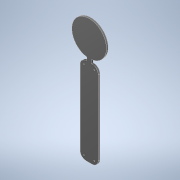
# Autodesk Inventor part: Body1
Saved by Autodesk Inventor 2022 (Build 260153000, 153)
## iProperties
Created: 2022-02-04
Part Number: Body1
Material: PVC-Piping
Document SubType Name: Modeling
Designer: joshw
Density: 1.4 g/cm^3
Appearance: Smooth - Black
Author: joshw
Autodesk Inventor part; units mm, degrees
ref_plane "YZ Plane" through (0, 0, 0) normal (1, 0, 0) x (0, 1, 0)
ref_plane "XZ Plane" through (0, 0, 0) normal (0, 1, 0) x (-1, 0, 0)
ref_plane "XY Plane" through (0, 0, 0) normal (0, 0, 1) x (1, 0, 0)
sketch "Sketch2" plane through (0, 0, 0) normal (0, 0, 1) x (1, 0, 0)
  line L0 (-4.7023, 28.2327) -> (-5.3373, 28.2327)
  line L1 (-5.3373, 28.2327) -> (-5.3373, 26.3277)
  line L2 (-4.7023, 26.3277) -> (-4.7023, 28.2327)
  line L3 (-5.3373, 26.3277) -> (-4.7023, 26.3277)
  arc A0 (-5.4629, 26.9627) -> (-6.3519, 26.0737) centre (-5.4629, 26.0737) ccw
  line L4 (-4.5766, 26.9627) -> (-5.4629, 26.9627)
  arc A1 (-3.6876, 26.0737) -> (-4.5766, 26.9627) centre (-4.5766, 26.0737) ccw
  line L5 (-3.6876, 15.1517) -> (-3.6876, 26.0737)
  arc A2 (-4.5766, 14.2627) -> (-3.6876, 15.1517) centre (-4.5766, 15.1517) ccw
  line L6 (-5.4629, 14.2627) -> (-4.5766, 14.2627)
  arc A3 (-6.3519, 15.1517) -> (-5.4629, 14.2627) centre (-5.4629, 15.1517) ccw
  line L7 (-6.3519, 26.0737) -> (-6.3519, 15.1517)
  line L8 (-6.3519, 14.2627) -> (-3.6876, 26.9627) construction
  line L9 (-3.6876, 14.2627) -> (-6.3519, 26.9627) construction
  line L10 (-5.3373, 26.3277) -> (-4.7023, 28.2327) construction
  line L11 (-4.7023, 26.3277) -> (-5.3373, 28.2327) construction
  circle A4 centre (-5.0198, 30.0107) radius 2.54
  circle A5 centre (-5.7772, 26.3881) radius 0.0635
  line L12 (-5.4629, 26.0737) -> (-6.0915, 26.7024) construction
  line L13 (-5.0198, 20.6127) -> (-3.948, 20.6127)
  line L14 (-3.948, 20.6127) -> (-5.0198, 20.6127)
  line L15 (-5.0198, 20.6127) -> (-5.0198, 22.4129)
  circle A6 centre (-4.2623, 26.3881) radius 0.0635
  circle A7 centre (-5.7772, 14.8374) radius 0.0635
  circle A8 centre (-4.2623, 14.8374) radius 0.0635
  point P0 (0, 0)
  point P1 (-5.3373, 26.9627)
  point P2 (-4.7023, 26.9627)
  point P3 (-4.7023, 27.4907)
  point P4 (-5.3373, 27.4907)
  dimension "d7" = 5.08
  dimension "d8" = 3.048
  dimension "d9" = 0.127
  dimension "d10" = 0.4445
  constraints: 32 end point, 9 centre point, 9 point on circle, 3 horizontal, 3 symmetric about line, 2 midpoint, 1 collinear, 1 vertical, 23 other
  measures "d7" diameter of A4
  measures "d8" distance from line of L4 A4.centre
  measures "d9" diameter of A5
  measures "d10" distance of A5.centre L12.start
extrude "Extrusion1" add sketch "Sketch2" along normal mid plane 0.254
body "Solid1"
